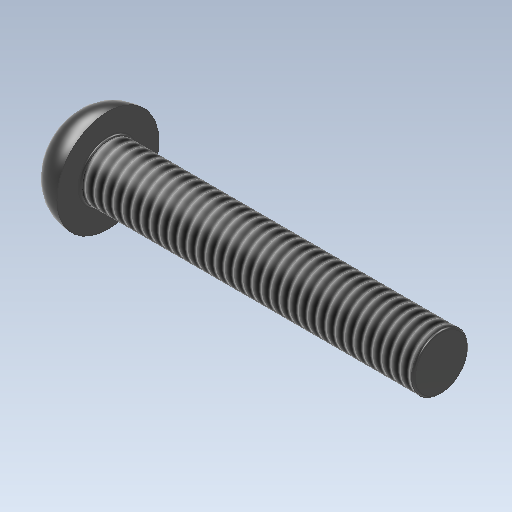
# Autodesk Inventor part: ネジボタンM3L18
Saved by Autodesk Inventor 2020.2 (Build 242310000, 310)
## iProperties
Created: 2020-02-24
Part Number: ネジボタンM3L18
Material: 鋼
Document SubType Name: Modeling
Designer: aoyam
Density: 7.85 g/cm^3
Appearance: サテン - 黒
Mass: 1.24354 g
Surface Area: 2.44037 cm^2
Volume: 0.158413 cm^3
Author: aoyam
Autodesk Inventor part; units mm, degrees
ref_plane "YZ Plane" through (0, 0, 0) normal (1, 0, 0) x (0, 1, 0)
ref_plane "XZ Plane" through (0, 0, 0) normal (0, 1, 0) x (-1, 0, 0)
ref_plane "XY Plane" through (0, 0, 0) normal (0, 0, 1) x (1, 0, 0)
sketch "スケッチ1" plane through (0, 0, 0) normal (0, 0, 1) x (1, 0, 0)
  line L0 (0, 0) -> (18, 0)
  line L1 (18, 0) -> (18, 1.5)
  line L2 (18, 1.5) -> (0, 1.5)
  line L3 (0, 1.5) -> (0, 0)
  line L4 (0, 0) -> (0, 2.75)
  line L5 (0, 0) -> (-2, 0)
  line L6 (-2, 0) -> (0, 0)
  line L7 (-2, 0) -> (-2, 1.15)
  arc A0 (0, 2.75) -> (-2, 1.15) centre (-0.0403, 0.7504) ccw
  dimension "d0" = 1.5
  dimension "d1" = 18
  dimension "d3" = 2
  dimension "d4" = 2.75
  dimension "d5" = 1.15
  dimension "d6" = 2
  constraints: 16 end point, 2 horizontal, 2 parallel, 2 point on circle, 2 vertical, 1 centre point, 1 perpendicular
  measures "d0" distance of L1.end L0.end
  measures "d1" distance of L1.end L2.end
  measures "d3" distance of L0.start L5.end
  measures "d4" distance of L0.start L4.end
  measures "d5" distance of L5.end L7.end
  measures "d6" radius of A0
revolve "回転1" add sketch "スケッチ1" angle 360 about axis through (-2, 0, 0) along (1, 0, 0)
thread "ねじ1" size "M3x0.5" class "6g" standard "ANSI Metric M Profile" length 100
sketch "スケッチ2" plane through (-2, 0, 0) normal (-1, 0, 0) x (0, 0, 1)
  circle A0 centre (0, 0) radius 1.15 projected
  line L0 (-0.575, 0.9959) -> (0.575, 0.9959)
  line L1 (0.575, 0.9959) -> (1.15, 0)
  line L2 (1.15, 0) -> (0.575, -0.9959)
  line L3 (0.575, -0.9959) -> (-0.575, -0.9959)
  line L4 (-0.575, -0.9959) -> (-1.15, 0)
  line L5 (-1.15, 0) -> (-0.575, 0.9959)
  dimension "d10" = 1.15
  dimension "d11" = 1.9919
  constraints: 12 end point, 1 coincident, 1 horizontal, 15 other
  measures "d10" distance of L0.start L0.end
  measures "d11" distance between parallel lines of L3 L0
extrude "押し出し1" cut sketch "スケッチ2" against normal blind 1.4 contours L2 L3 L4 L5 L0 L1
fillet "フィレット1" radius 0.2 6 edges at (-0.6, 0.9959, 0) (-0.6, 0.498, 0.8625) (-0.6, 0.498, -0.8625) (-0.6, -0.498, -0.8625) (-0.6, -0.9959, 0) (-0.6, -0.498, 0.8625)
fillet "フィレット2" radius 0.1 1 edges at (0, -1.5, 0)
fillet "フィレット3" radius 0.1 1 edges at (18, -1.5, 0)
